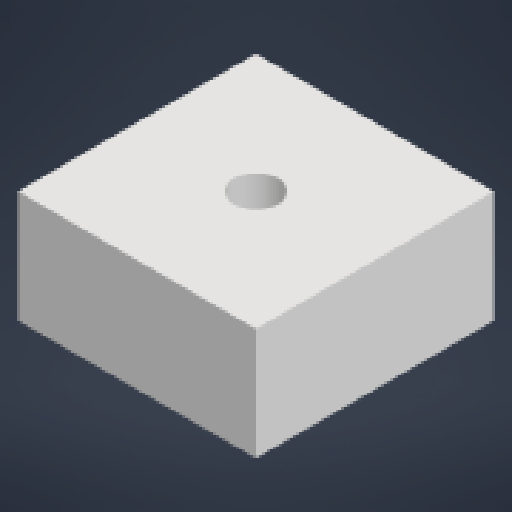
# Autodesk Inventor part: track
Saved by Autodesk Inventor 2023 (Build 270158000, 158)
## iProperties
Created: 2023-01-24
Part Number: track
Material: Generic
Document SubType Name: Modeling
Designer: Blank Slate
Density: 1 g/cm^3
Appearance: Default
Author: Blank Slate
Autodesk Inventor part; units mm, degrees
ref_plane "YZ Plane" through (0, 0, 0) normal (1, 0, 0) x (0, 1, 0)
ref_plane "XZ Plane" through (0, 0, 0) normal (0, 1, 0) x (-1, 0, 0)
ref_plane "XY Plane" through (0, 0, 0) normal (0, 0, 1) x (1, 0, 0)
sketch "Sketch1" plane through (0, 0, 0) normal (0, 1, 0) x (-1, 0, 0)
  line L0 (0, 0) -> (-228.6, 0)
  line L1 (-228.6, 0) -> (-228.6, -25.4)
  line L2 (-228.6, -25.4) -> (0, -25.4)
  line L3 (0, -25.4) -> (0, 0)
  dimension "d0" = 228.6
  dimension "d1" = 25.4
  constraints: 8 end point, 2 parallel, 1 horizontal, 1 perpendicular
  measures "d0" distance of L2.end L1.end
  measures "d1" distance of L1.end L0.end
extrude "Extrusion1" add sketch "Sketch1" along normal blind 11.938
sketch "Sketch4" plane through (0, 11.938, 0) normal (0, 1, 0) x (1, 0, 0)
  line L0 (228.6, 25.4) -> (0, 25.4) projected
  line L1 (114.3, 25.4) -> (114.3, 0) construction
  line L2 (0, 0) -> (228.6, 0) projected
  circle A0 centre (114.3, 12.7) radius 2.3812
  line L3 (0, 25.4) -> (0, 0) projected
  line L4 (0, 12.7) -> (12.7, 12.7)
  line L5 (0, 12.7) -> (12.7, 12.7) construction
  circle A1 centre (12.7, 12.7) radius 2.3812
  dimension "d40" = 12.7
  dimension "d42" = 4.7625
  constraints: 6 end point, 4 midpoint, 2 centre point, 2 horizontal, 1 coincident, 1 collinear
  measures "d40" distance of L4.start L4.end
  measures "d42" diameter of A1
hole "Hole3" at (114.3, 11.938, -12.7) at (12.7, 11.938, -12.7) direction (0, -1, 0) diameter 4.7625 end through all
body "Solid1"
